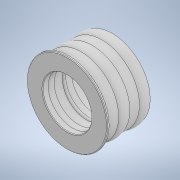
# Autodesk Inventor part: DustPortConvertorShort
Saved by Autodesk Inventor 2022 (Build 260153000, 153)
## iProperties
Created: 2021-11-07
Part Number: DustPortConvertorShort
Material: Generic
Document SubType Name: Modeling
Designer: dangl
Density: 1 g/cm^3
Appearance: Default
Author: dangl
Autodesk Inventor part; units mm, degrees
ref_plane "YZ Plane" through (0, 0, 0) normal (1, 0, 0) x (0, 1, 0)
ref_plane "XZ Plane" through (0, 0, 0) normal (0, 1, 0) x (-1, 0, 0)
ref_plane "XY Plane" through (0, 0, 0) normal (0, 0, 1) x (1, 0, 0)
sketch "Sketch1" plane through (0, 0, 0) normal (0, 1, 0) x (-1, 0, 0)
  line L0 (0, 0) -> (0, -30)
  line L1 (0, 0) -> (-28.5, 0)
  line L2 (-28.5, -35) -> (-25.5, -35)
  line L3 (-25.5, -35) -> (-18, -25)
  line L4 (-18, -25) -> (-18.1552, -17.2395)
  arc A0 (-18.1552, -17.2395) -> (-18.2054, -14.7277) centre (-19, -16) ccw
  line L5 (-18.2054, -14.7277) -> (-18.326, -8.6999)
  line L6 (-30.5, 0) -> (-30.5, -2)
  line L7 (-30.5, -2) -> (-28.75, -2)
  line L8 (-28.5, 0) -> (-30.5, 0)
  line L9 (-28.5, -2.25) -> (-28.5, -9.6047)
  arc A1 (-28.5, -2.25) -> (-28.75, -2) centre (-28.75, -2.25) ccw
  arc A2 (-18.326, -8.6999) -> (-18.4158, -4.2121) centre (-25, -6.5886) ccw
  line L10 (-18.4158, -4.2121) -> (-18.5, 0)
  arc A3 (-28.5, -26.5147) -> (-28.5, -35) centre (-20, -30.7574) ccw
  arc A4 (-28.5, -10.7574) -> (-28.5, -19.2426) centre (-20, -15) ccw
  line L11 (-28.5, -10.7574) -> (-28.5, -9.6047)
  line L12 (-28.5, -26.5147) -> (-28.5, -19.2426)
  dimension "d0" = 30
  dimension "d13" = 3
  dimension "d14" = 25
  dimension "d15" = 35
  dimension "d16" = 18
  dimension "d17" = 18.5
  dimension "d25" = 16
  dimension "d26" = 19
  dimension "d27" = 3
  dimension "d32" = 2
  dimension "d33" = 2
  dimension "d34" = 0.25
  dimension "d37" = 25
  dimension "d43" = 20
  dimension "d45" = 15
  dimension "d46" = 20
  constraints: 26 end point, 10 point on circle, 5 centre point, 4 vertical, 2 collinear, 2 horizontal, 2 tangent, 1 perpendicular, 1 point on line
  measures "d0" distance of L0.start L0.end
  measures "d13" distance of L2.start L2.end
  measures "d14" vertical distance of L0.start L3.end
  measures "d15" distance between parallel lines of L1 L2
  measures "d16" distance from line of L0 L3.end
  measures "d17" distance of L0.start L10.end
  measures "d25" vertical distance of L0.start A0.centre
  measures "d26" distance from line of L0 A0.centre
  measures "d27" diameter of A0
  measures "d32" distance between parallel lines of L8 L7
  measures "d33" distance from line of L1.end L6
  measures "d34" radius of A1
  measures "d37" distance from line of L0 A2.centre
  measures "d43" horizontal distance of L0.start A3.centre
  measures "d45" vertical distance of L0.start A4.centre
  measures "d46" horizontal distance of L0.start A4.centre
revolve "Revolution1" add sketch "Sketch1" angle 360 about axis through (0, 0, 0) along (0, 0, -1)
fillet "Fillet1" radius 0.5 1 edges at (-18.5, 0, 0)
fillet "Fillet2" radius 2 1 edges at (-25.5, 0, -35)
fillet "Fillet3" radius 1 1 edges at (-28.5, 0, -35)
fillet "Fillet4" radius 0.5 2 edges at (-30.5, 0, -2) (-30.5, 0, 0)
fillet "Fillet5" radius 10 1 edges at (-18, 0, -25)
equation "\"d46\" = d43"
body "Solid1"
